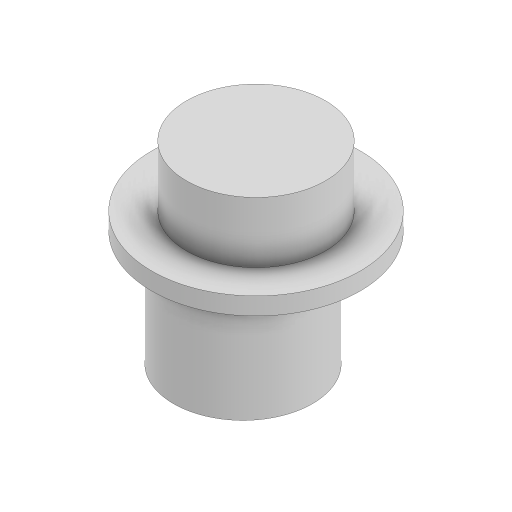
# Autodesk Inventor part: Dysk_we
Saved by Autodesk Inventor 2024 (Build 280153000, 153)
## iProperties
Created: 2024-12-22
Part Number: Dysk_we
Material: Ogólny
Document SubType Name: Modeling
Designer: Wicek
Density: 1 g/cm^3
Appearance: Domyślna
Lrz: 11,000 mm
Lrw: 4,000 mm
Lh: 7,000 mm
N1: 31,000 ul
Rr: 1,500 mm
R: 29,603 mm
R1: 5,000 mm
h1: 2,000 mm
h2: 5,000 mm
E1: 0,750 mm
dwr1: 4,276 mm
dwr2: 20,301 mm
dwr: 29,603 mm
Author: Wicek
Autodesk Inventor part; units mm, degrees
ref_plane "YZ Plane" through (0, 0, 0) normal (1, 0, 0) x (0, 1, 0)
ref_plane "XZ Plane" through (0, 0, 0) normal (0, 1, 0) x (-1, 0, 0)
ref_plane "XY Plane" through (0, 0, 0) normal (0, 0, 1) x (1, 0, 0)
sketch "Szkic1" plane through (0, 0, 0) normal (0, 1, 0) x (-1, 0, 0)
  circle A0 centre (0, 0) radius 4
  arc A1 (-2.25, -2) -> (-2.25, 2) centre (-0.75, 0) ccw
  line L0 (-2.25, 2) -> (-2.25, -2)
  dimension "d2" = 4
  dimension "d15" = 2.5
  dimension "d16" = 0.75
  dimension "d23" = 1.5
  constraints: 2 centre point, 2 end point, 2 point on circle, 1 coincident, 1 vertical
  measures "d2" radius of A0
  measures "d15" radius of A1
  measures "d16" distance of A0.centre A1.centre
  measures "d23" distance from line of L0 A1.centre
extrude "Wyciągnięcie proste1" add sketch "Szkic1" along normal blind 7
sketch "Szkic2" plane through (0, 7, 0) normal (0, 1, 0) x (1, 0, 0)
  circle A0 centre (0.75, 0) radius 6
  arc A1 (2.25, 2) -> (2.25, -2) centre (0.75, 0) ccw projected
  arc A2 (2.25, 2) -> (2.25, -2) centre (0.75, 0) ccw projected
  dimension "d32" = 6
  constraints: 2 coincident, 1 centre point
  measures "d32" radius of A0
extrude "Wyciągnięcie proste2" add sketch "Szkic2" along normal blind 1
sketch "Szkic3" plane through (0.75, 8, 0) normal (0, 1, 0) x (1, 0, 0)
  circle A0 centre (0, 0) radius 4
  circle A1 centre (0, 0) radius 6 projected
  arc A2 (1.5, 2) -> (1.5, -2) centre (0, 0) ccw projected
  dimension "d33" = 4
  constraints: 2 coincident, 1 centre point
  measures "d33" radius of A0
extrude "Wyciągnięcie proste3" add sketch "Szkic3" along normal blind 3.5 contours A0
equation "\"d2\" = Lrw"
equation "\"d15\" = silnik_rw"
equation "\"d16\" = E1"
equation "\"d28\" = Lh"
equation "\"d33\" = Lrw"
equation "\"d34\" = 0.5 * Lh"
equation "\"Lrz\" = 11"
equation "\"Lrw\" = 4"
equation "\"Lh\" = 7"
equation "\"N1\" = 31"
equation "\"Rr\" = 1.5"
equation "\"R1\" = 5"
equation "\"h1\" = 2"
equation "\"h2\" = 5"
equation "\"E1\" = 0.5 * Rr"
equation "\"dwr1\" = -0.25 * Rr + 0.25 * R - 0.25 * Lrz"
equation "\"dwr2\" = 0.5 * Lrz + 0.5 * R"
equation "\"dwr\" = R"
equation "\"silnik_rw\" = 2.5"
equation "\"silnik_r_wypust\" = Lrz"
equation "\"silnik_d_srub\" = 31"
equation "\"R\" = 29.602819"
